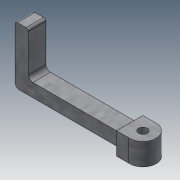
# Autodesk Inventor part: J007872 GRIN LENS HOLDER 0_5MM DIA Rev -
Saved by Autodesk Inventor 2018.3 (Build 223284000, 284)
## iProperties
Created: 2019-01-28
Material: STAINLESS STEEL, 316
Vendor: HHMI: JRC - ID&F
Document SubType Name: Modeling
Designer: arnoldj
Density: 8 g/cm^3
Appearance: Metal-Steel (Stainless, Brushed)
Part Number: J007872 GRIN LENS HOLDER 0_5MM DIA Rev -
Project: COMMON
Description: GRIN LENS HOLDER 0_5MM DIA
RuleStatus: InUse
AfterDocSave0: file://Part Number Cleaner
LAB/DEPT: STERNSON (LAB)
REQUESTING SCIENTIST: COMMON
SURFACE ROUGHNESS: 63 Ra
DESIGN DEPARTMENT: HHMI: JRC - ID&F
SPECIAL FINISH: NONE
ALTERED ITEM PART NUMBER: N/A
ALTERED ITEM VENDOR: N/A
ALTERED ITEM DESCRIPTION: N/A
Author: arnoldj
Revision Number: -
Autodesk Inventor part; units mm, degrees
ref_plane "YZ Plane" through (0, 0, 0) normal (1, 0, 0) x (0, 1, 0)
ref_plane "XZ Plane" through (0, 0, 0) normal (0, 1, 0) x (-1, 0, 0)
ref_plane "XY Plane" through (0, 0, 0) normal (0, 0, 1) x (1, 0, 0)
sketch "Sketch1" plane through (0, 0, 0) normal (0, 0, 1) x (1, 0, 0)
  line L0 (0, 4.0132) -> (0, -0.9652) projected
  line L1 (-1.524, 0) -> (9.144, 0) projected
  line L2 (7.62, 0) -> (0, 0)
  line L3 (0, 0) -> (0, 0.762)
  line L4 (0, 0.762) -> (7.62, 0.762)
  line L5 (7.62, 0.762) -> (7.62, 0)
  line L6 (0, 0.762) -> (0.762, 0.762)
  line L7 (0.762, 0.762) -> (0.762, 3.302)
  line L8 (0.762, 3.302) -> (0, 3.302)
  line L9 (0, 3.302) -> (0, 0.762)
  line L10 (6.096, -0.254) -> (7.62, -0.254)
  line L11 (7.62, -0.254) -> (7.62, 1.016)
  line L12 (7.62, 1.016) -> (6.096, 1.016)
  line L13 (6.096, 1.016) -> (6.096, -0.254)
  line L14 (6.096, -0.254) -> (7.62, 1.016) construction
  line L15 (7.62, -0.254) -> (6.096, 1.016) construction
  line L16 (0, 0.381) -> (7.62, 0.381) construction
  point P0 (6.858, 0.381)
  dimension "d0" = 0.762
  dimension "d1" = 0.762
  dimension "d2" = 3.302
  dimension "d4" = 1.27
  dimension "d5" = 1.524
  dimension "d6" = 6.858
  dimension "d7" = 0
  constraints: 30 end point, 6 parallel, 4 midpoint, 4 perpendicular, 3 horizontal, 2 point on line, 1 vertical alignment
  measures "d0" distance of L7.end L8.end
  measures "d1" distance of L4.end L2.start
  measures "d2" distance between parallel lines of L1 L8
  measures "d4" distance of L12.end L10.start
  measures "d5" distance of L11.end L12.end
  measures "d6" distance from line of L0 point (6.858, 0.381)
  measures "d7" distance from line of L16 point (6.858, 0.381)
extrude "Extrusion1" add sketch "Sketch1" along normal mid plane 1.016 contours L8 L7 L4 L0 | L4 L13 L1 L0 | L13 L4 L5 L1
sketch "Sketch2" plane through (0.762, 0.762, 0.508) normal (0, 1, 0) x (1, 0, 0)
  line L0 (-0.762, 1.5748) -> (-0.762, -0.5588) projected
  line L1 (8.382, 0.508) -> (-2.286, 0.508) projected
  line L2 (6.858, 1.016) -> (6.858, 0) projected
  circle A0 centre (6.096, 0.508) radius 0.762
  line L3 (0, 1.016) -> (6.858, 1.016) projected
  line L4 (6.858, 0) -> (0, 0) projected
  line L5 (6.664, 0) -> (6.858, 0)
  line L6 (6.858, 0) -> (6.858, 1.016)
  line L7 (6.858, 1.016) -> (6.664, 1.016)
  line L8 (5.334, -0.2504) -> (6.0218, -0.2504)
  line L9 (6.0218, -0.2504) -> (6.0218, 1.2664)
  line L10 (6.0218, 1.2664) -> (5.334, 1.2664)
  line L11 (5.334, 1.2664) -> (5.334, -0.2504)
  line L12 (5.334, -0.2504) -> (6.0218, 1.2664) construction
  line L13 (6.0218, -0.2504) -> (5.334, 1.2664) construction
  point P0 (-0.762, 0.508)
  point P1 (5.6779, 0.508)
  dimension "d10" = 1.524
  dimension "d30" = 6.096
  constraints: 18 end point, 4 point on line, 3 equal length, 3 point on circle, 2 horizontal, 2 midpoint, 1 centre point, 1 perpendicular, 1 tangent
  measures "d10" diameter of A0
  measures "d30" distance between parallel lines of L11 L0
extrude "Extrusion2" add sketch "Sketch2" against normal blind 1.016 and the other way blind 0.254 contours A0 L4 L9 L1 | L1 L9 L3 A0 | L9 L4 A0 L1 | L1 A0 L3 L9 | L3 L9 A0 | A0 L9 L4 | L11 L3 A0 | A0 L4 L11 | L9 A0 L4 | L3 A0 L9 | A0 L3 L11 L10 | L8 L11 L4 A0
extrude "Extrusion3" cut sketch "Sketch2" against normal up to next contours A0 L3 L2 | L2 L4 A0
hole "Hole1" at (6.858, 1.016, 0) direction (0, -1, 0) diameter 0.508 end through all
fillet "Fillet2" radius 0.254 2 edges at (0.762, 0.762, 0) (0, 0, 0)
fillet "Fillet3" radius 0.127 2 edges at (6.096, 0.381, 0.508) (6.096, 0.381, -0.508)
fillet "Fillet4" radius 0.127 2 edges at (0, 3.302, 0) (0.762, 3.302, 0)
body "Solid1"
